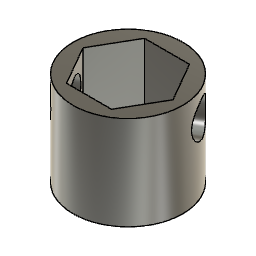
manivela (Autodesk Fusion 360 design; units mm, degrees)
Autodesk Fusion 360 part; units mm, degrees
sketch "Boceto1" plane through (0, 0, 0) normal (0, 0, 1) x (1, 0, 0)
  circle A0 centre (0, 0) radius 11.5
  line L0 (0, 0) -> (11.5, 0)
  line L1 (0, 0) -> (5.75, 9.9593)
  line L2 (0, 0) -> (-5.75, 9.9593)
  line L3 (0, 0) -> (-11.5, 0)
  line L4 (0, 0) -> (-5.75, -9.9593)
  line L5 (0, 0) -> (5.75, -9.9593)
  line L6 (5.75, 9.9593) -> (-5.75, 9.9593)
  line L7 (-5.75, 9.9593) -> (-11.5, 0)
  line L8 (-11.5, 0) -> (-5.75, -9.9593)
  line L9 (-5.75, -9.9593) -> (5.75, -9.9593)
  line L10 (5.75, -9.9593) -> (11.5, 0)
  line L11 (11.5, 0) -> (5.75, 9.9593)
  circle A1 centre (0, 0) radius 14
  dimension "d1" = 23
  dimension "d3" = 360
  dimension "d5" = 360
  dimension "d6" = 28
  constraint coincident A0.centre L0.start
  constraint coincident A0 L0.end
  constraint horizontal L0
  constraint concentric A0 A1
  measures "d1" diameter of A0
  measures "d6" diameter of A1
extrude "Extruir1" add sketch "Boceto1" along normal blind 24 contours A0 L11 | A0 L10 | A0 L6 | A0 L9 | A0 L7 | A0 L8 | A1
sketch "Boceto2" plane through (8.625, 4.9796, 0) normal (-0.866025, -0.5, 0) x (0.5, -0.866025, 0)
  line L0 (-5.75, 0) -> (5.75, 0)
  line L1 (5.75, 0) -> (5.75, 24)
  line L2 (5.75, 24) -> (-5.75, 24)
  line L3 (-5.75, 24) -> (-5.75, 0)
  circle A0 centre (0.25, 17) radius 4.5
  dimension "d9" = 9
  dimension "d10" = 7
  dimension "d11" = 5.5
  measures "d9" diameter of A0
  measures "d10" distance of L2 A0.centre
  measures "d11" distance of L1 A0.centre
extrude "Extruir2" cut sketch "Boceto2" along normal mid plane 54 contours A0
